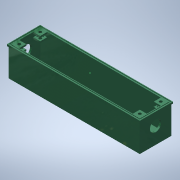
# Autodesk Inventor part: base inferior
Saved by Autodesk Inventor 2021 (Build 250183000, 183)
## iProperties
Created: 2021-03-08
Part Number: base inferior
Material: Steel, Mild, Welded
Document SubType Name: Modeling
Designer: Usuario
Density: 7.85 g/cm^3
Appearance: Smooth - Dark Sea Green
Author: Usuario
Autodesk Inventor part; units mm, degrees
ref_plane "YZ Plane" through (0, 0, 0) normal (1, 0, 0) x (0, 1, 0)
ref_plane "XZ Plane" through (0, 0, 0) normal (0, 1, 0) x (-1, 0, 0)
ref_plane "XY Plane" through (0, 0, 0) normal (0, 0, 1) x (1, 0, 0)
sketch "Sketch1" plane through (0, 0, 0) normal (0, 1, 0) x (-1, 0, 0)
  line L0 (75, -18) -> (-75, -18)
  line L1 (-75, -18) -> (-75, 18)
  line L2 (-75, 18) -> (75, 18)
  line L3 (75, 18) -> (75, -18)
  line L4 (75, -18) -> (-75, 18) construction
  line L5 (-75, -18) -> (75, 18) construction
  point P0 (0, 0)
  dimension "d0" = 150
  dimension "d1" = 36
  constraints: 12 end point, 2 midpoint, 2 parallel, 1 horizontal, 1 perpendicular
  measures "d0" distance of L1.end L2.end
  measures "d1" distance of L0.end L1.end
extrude "Extrusion1" add sketch "Sketch1" along normal blind 2
sketch "Sketch3" plane through (0, 2, 0) normal (0, 1, 0) x (1, 0, 0)
  line L0 (75, 18) -> (-75, 18) projected
  line L1 (-75, 18) -> (-75, -18) projected
  line L2 (73, -16) -> (-73, -16)
  line L3 (-73, -16) -> (-73, 16)
  line L4 (-73, 16) -> (73, 16)
  line L5 (73, 16) -> (73, -16)
  line L6 (-75, -18) -> (75, -18) projected
  line L7 (-75, -18) -> (75, -18)
  line L8 (75, -18) -> (75, 18)
  line L9 (75, 18) -> (-75, 18)
  line L10 (-75, 18) -> (-75, -18)
  point P0 (0, 0)
  constraints: 16 end point, 4 parallel, 2 horizontal, 2 perpendicular
extrude "Extrusion3" add sketch "Sketch3" along normal blind 30
sketch "Sketch4" plane through (-73, 2, 16) normal (1, 0, 0) x (0, 0, -1)
  line L0 (32, 0) -> (0, 0) projected
  line L1 (32, 0) -> (32, 30) projected
  line L2 (0, 30) -> (32, 30) projected
  line L3 (0, 0) -> (0, 30) projected
  line L4 (0, 30) -> (32, 30) projected
  line L5 (32, 0) -> (32, 30) projected
  line L6 (0, 30) -> (32, 30)
  line L7 (32, 30) -> (32, 0)
  line L8 (32, 0) -> (0, 0)
  line L9 (0, 0) -> (0, 30)
  line L10 (32, 0) -> (0, 0) projected
  circle A0 centre (16, 17) radius 6.4
  point P0 (16, -2)
  constraints: 8 end point, 2 parallel, 1 centre point, 1 horizontal, 1 perpendicular
extrude "Extrusion4" cut sketch "Sketch4" against normal blind 30 contours A0
sketch "Sketch5" plane through (73, 2, -16) normal (-1, 0, 0) x (0, 0, 1)
  line L0 (32, 0) -> (0, 0) projected
  line L1 (32, 0) -> (32, 30) projected
  line L2 (0, 30) -> (32, 30) projected
  line L3 (0, 0) -> (0, 30) projected
  line L4 (0, 30) -> (32, 30) projected
  line L5 (0, 30) -> (32, 30)
  line L6 (32, 30) -> (32, 0)
  line L7 (32, 0) -> (0, 0)
  line L8 (0, 0) -> (0, 30)
  line L9 (0, 0) -> (0, 30) projected
  circle A0 centre (16, 17) radius 6.4
  point P0 (16, -2)
  dimension "d23" = 12.8
  constraints: 8 end point, 2 parallel, 1 centre point, 1 horizontal, 1 perpendicular
  measures "d23" diameter of A0
extrude "Extrusion5" cut sketch "Sketch5" against normal blind 30 contours A0
sketch "Sketch6" plane through (0, 32, 0) normal (0, 1, 0) x (1, 0, 0)
  line L0 (75, 18) -> (-75, 18) projected
  line L1 (-75, 18) -> (-75, -18) projected
  line L2 (-75, -18) -> (75, -18) projected
  line L3 (75, -18) -> (75, 18) projected
  line L4 (73, -16) -> (-73, -16) projected
  line L5 (-73, -16) -> (-73, 16) projected
  line L6 (-73, 16) -> (73, 16) projected
  line L7 (73, 16) -> (73, -16) projected
  line L8 (-76, -18) -> (-76, -19)
  line L9 (75, -18) -> (75, 18) projected
  line L10 (75, 19) -> (76, 19)
  line L11 (76, 19) -> (-76, 19)
  line L12 (-76, 19) -> (-76, -19)
  line L13 (-76, -19) -> (76, -19)
  line L14 (76, -19) -> (76, 19)
  line L15 (-73, -16) -> (-73, 16) projected
  line L16 (73, 16) -> (-73, 16) projected
  line L17 (-73, -16) -> (73, -16)
  line L18 (73, -16) -> (73, 16)
  line L19 (73, 16) -> (-73, 16)
  line L20 (-73, 16) -> (-73, -16)
  point P0 (0, 0)
  dimension "d26" = 1
  dimension "d27" = 1
  dimension "d28" = 1
  dimension "d29" = 1
  constraints: 20 end point, 4 parallel, 2 horizontal, 2 perpendicular
  measures "d26" distance of L1.end L8.start
  measures "d27" distance of L8.start L8.end
  measures "d28" distance of L0.start L10.start
  measures "d29" distance of L10.start L10.end
extrude "Extrusion6" add sketch "Sketch6" along normal blind 2 contours L3 L2 L1 L0 | L12 L11 L10 L14 L13 L8
sketch "Sketch7" plane through (0, 34, 0) normal (0, 1, 0) x (1, 0, 0)
  line L0 (76, 19) -> (-76, 19) projected
  line L1 (-76, 19) -> (-76, -19) projected
  line L2 (-76, -19) -> (76, -19) projected
  line L3 (76, -19) -> (76, 19) projected
  line L4 (73, 16) -> (73, -16) projected
  line L5 (73, -16) -> (-73, -16) projected
  line L6 (-73, -16) -> (-73, 16) projected
  line L7 (-73, 16) -> (73, 16) projected
  line L8 (73, -16) -> (-73, -16) projected
  line L9 (-73.85, -16) -> (-73.85, -16.85)
  line L10 (-76, 19) -> (-76, -19) projected
  line L11 (-76, -19) -> (-76, -18.15)
  line L12 (76, 19) -> (-76, 19) projected
  line L13 (76, 19) -> (75.15, 19)
  line L14 (-73, 16) -> (73, 16) projected
  line L15 (73, 16.85) -> (73.85, 16.85)
  line L16 (73.85, 16.85) -> (-73.85, 16.85)
  line L17 (-73.85, 16.85) -> (-73.85, -16.85)
  line L18 (-73.85, -16.85) -> (73.85, -16.85)
  line L19 (73.85, -16.85) -> (73.85, 16.85)
  line L20 (-75.15, -18.15) -> (75.15, -18.15)
  line L21 (75.15, -18.15) -> (75.15, 18.15)
  line L22 (75.15, 18.15) -> (-75.15, 18.15)
  line L23 (-75.15, 18.15) -> (-75.15, -18.15)
  point P0 (0, 0)
  dimension "d34" = 0.85
  constraints: 24 end point, 4 parallel, 2 horizontal, 2 perpendicular, 2 point on line
  measures "d34" distance of L1.end L11.end
extrude "Extrusion7" cut sketch "Sketch7" against normal blind 0.75 contours L23 L22 L21 L20
sketch "Sketch8" plane through (0, 34, 0) normal (0, 1, 0) x (1, 0, 0)
  point P0 (0, 0)
sketch "Sketch9" plane through (-73, 2, 16) normal (1, 0, 0) x (0, 0, -1)
  point P0 (16, -2)
sketch "Sketch29" plane through (0, 34, 0) normal (0, 1, 0) x (1, 0, 0)
  line L0 (-73.85, -16.85) -> (73.85, -16.85) projected
  line L1 (73.85, -16.85) -> (73.85, 16.85) projected
  line L2 (73.85, 16.85) -> (-73.85, 16.85) projected
  line L3 (-73.85, 16.85) -> (-73.85, -16.85) projected
  line L4 (73, 16) -> (73, -16) projected
  line L5 (73, -16) -> (-73, -16) projected
  line L6 (-73, -16) -> (-73, 16) projected
  line L7 (-73, 16) -> (73, 16) projected
  line L8 (75.15, 18.15) -> (75.15, -18.15) projected
  line L9 (-75.15, 18.15) -> (75.15, 18.15) projected
  line L10 (-75.15, -18.15) -> (-75.15, 18.15) projected
  line L11 (75.15, -18.15) -> (-75.15, -18.15) projected
  line L12 (73.85, -16.85) -> (73.85, 16.85) projected
  line L13 (-73.85, -16.85) -> (73.85, -16.85) projected
  line L14 (-73.85, 16.85) -> (-73.85, -16.85) projected
  line L15 (73.85, 16.85) -> (-73.85, 16.85) projected
  line L16 (-76, 19) -> (-76, -19) projected
  line L17 (76, 19) -> (-76, 19) projected
  line L18 (-76, 19) -> (-76, -19) projected
  line L19 (-76, -19) -> (76, -19) projected
  line L20 (76, -19) -> (76, 19) projected
  line L21 (-75.15, 18.15) -> (75.15, 18.15) projected
  line L22 (75.15, 18.15) -> (75.15, -18.15) projected
  line L23 (75.15, -18.15) -> (-75.15, -18.15) projected
  line L24 (-75.15, -18.15) -> (-75.15, 18.15) projected
  line L25 (-73, -16) -> (73, -16) projected
  line L26 (-73, -16) -> (-73, 16) projected
  line L27 (-73, -16) -> (-65.5, -16) construction
  line L28 (-73, -16) -> (-65, -16)
  line L29 (-65, -16) -> (-65, -8)
  line L30 (-65, -8) -> (-73, -8)
  line L31 (-73, -8) -> (-73, -16)
  line L32 (-73, 16) -> (-65, 16)
  line L33 (-65, 16) -> (-65, 8)
  line L34 (-65, 8) -> (-73, 8)
  line L35 (-73, 8) -> (-73, 16)
  line L36 (73, 16) -> (-73, 16) projected
  line L37 (73, 16) -> (65, 16)
  line L38 (65, 16) -> (65, 8)
  line L39 (65, 8) -> (73, 8)
  line L40 (73, 8) -> (73, 16)
  line L41 (73, -16) -> (65, -16)
  line L42 (65, -16) -> (65, -8)
  line L43 (65, -8) -> (73, -8)
  line L44 (73, -8) -> (73, -16)
  point P0 (0, 0)
  dimension "d120" = 8
  dimension "d121" = 8
  dimension "d122" = 8
  dimension "d123" = 8
  dimension "d124" = 8
  dimension "d125" = 8
  dimension "d126" = 8
  dimension "d127" = 8
  constraints: 34 end point, 8 parallel, 5 horizontal, 4 perpendicular
  measures "d120" distance of L30.end L29.end
  measures "d121" distance of L29.end L28.end
  measures "d122" distance of L33.end L34.end
  measures "d123" distance of L32.end L33.end
  measures "d124" distance of L39.end L38.end
  measures "d125" distance of L38.end L37.end
  measures "d126" distance of L42.end L43.end
  measures "d127" distance of L41.end L42.end
extrude "Extrusion22" add sketch "Sketch29" against normal blind 7 contours L4 L39 L38 L7 | L4 L5 L42 L43 | L33 L34 L6 L7 | L5 L6 L30 L29
sketch "Sketch30" plane through (-65, 34, -8) normal (1, 0, 0) x (0, 0, -1)
  line L0 (0, 0) -> (8, 0) projected
  line L1 (0, 0) -> (0, -7) projected
  line L2 (8, -7) -> (0, -7) projected
  line L3 (8, 0) -> (8, -7) projected
  line L4 (-24, 0) -> (-16, 0) projected
  line L5 (-24, -7) -> (-24, 0) projected
  line L6 (-16, -7) -> (-24, -7) projected
  line L7 (-16, 0) -> (-16, -7) projected
  line L8 (0, 0) -> (0, -7) projected
  line L9 (8, 0) -> (0, 0)
  line L10 (0, 0) -> (0, -1.8)
  line L11 (0, -1.8) -> (8, -1.8)
  line L12 (8, -1.8) -> (8, 0)
  line L13 (8, 0) -> (8, -7) projected
  line L14 (8, -7) -> (0, -7)
  line L15 (0, -7) -> (0, -5.2)
  line L16 (0, -5.2) -> (8, -5.2)
  line L17 (8, -5.2) -> (8, -7)
  line L18 (0, -1.8) -> (8, -1.8)
  line L19 (8, -1.8) -> (8, -5.2)
  line L20 (8, -5.2) -> (0, -5.2)
  line L21 (0, -5.2) -> (0, -1.8)
  line L22 (-24, 0) -> (-16, 0) projected
  line L23 (-16, 0) -> (-24, 0)
  line L24 (-24, 0) -> (-24, -1.8)
  line L25 (-24, -1.8) -> (-16, -1.8)
  line L26 (-16, -1.8) -> (-16, 0)
  line L27 (-16, -7) -> (-24, -7)
  line L28 (-24, -7) -> (-24, -5.2)
  line L29 (-24, -5.2) -> (-16, -5.2)
  line L30 (-16, -5.2) -> (-16, -7)
  line L31 (-16, -1.8) -> (-24, -1.8)
  line L32 (-24, -1.8) -> (-24, -5.2)
  line L33 (-24, -5.2) -> (-16, -5.2)
  line L34 (-16, -5.2) -> (-16, -1.8)
  point P0 (-8, -34)
  point P1 (-24, -5.2)
  point P2 (-16, -5.2)
  point P3 (-16, -1.8)
  point P4 (-24, -1.8)
  point P5 (0, -5.2)
  point P6 (8, -5.2)
  point P7 (8, -1.8)
  point P8 (0, -1.8)
  dimension "d130" = 1.8
  dimension "d131" = 1.8
  dimension "d132" = 8
  dimension "d133" = 1.8
  dimension "d134" = 8
  dimension "d135" = 1.8
  constraints: 48 end point, 12 parallel, 6 horizontal, 6 perpendicular, 2 point on line
  measures "d130" distance of L10.end L9.end
  measures "d131" distance of L14.end L15.end
  measures "d132" distance of L25.end L24.end
  measures "d133" distance of L24.end L23.end
  measures "d134" distance of L28.end L29.end
  measures "d135" distance of L27.end L28.end
extrude "Extrusion23" cut sketch "Sketch30" against normal blind 8 contours L11 L3 L16 L1 | L25 L7 L29 L5
sketch "Sketch31" plane through (65, 34, -16) normal (-1, 0, 0) x (0, 0, 1)
  point P0 (16, -34)
sketch "Sketch32" plane through (65, 34, -16) normal (-1, 0, 0) x (0, 0, 1)
  line L0 (0, 0) -> (8, 0) projected
  line L1 (0, -7) -> (0, 0) projected
  line L2 (8, -7) -> (0, -7) projected
  line L3 (8, 0) -> (8, -7) projected
  line L4 (32, -7) -> (24, -7) projected
  line L5 (24, 0) -> (32, 0) projected
  line L6 (24, 0) -> (24, -7) projected
  line L7 (32, -7) -> (24, -7) projected
  line L8 (32, 0) -> (32, -7) projected
  line L9 (0, 0) -> (8, 0)
  line L10 (8, 0) -> (8, -1.8)
  line L11 (8, -1.8) -> (0, -1.8)
  line L12 (0, -1.8) -> (0, 0)
  line L13 (8, -7) -> (0, -7)
  line L14 (0, -7) -> (0, -5.2)
  line L15 (0, -5.2) -> (8, -5.2)
  line L16 (8, -5.2) -> (8, -7)
  line L17 (0, -1.8) -> (8, -1.8)
  line L18 (8, -1.8) -> (8, -5.2)
  line L19 (8, -5.2) -> (0, -5.2)
  line L20 (0, -5.2) -> (0, -1.8)
  line L21 (24, 0) -> (32, 0) projected
  line L22 (24, 0) -> (32, 0)
  line L23 (32, 0) -> (32, -1.8)
  line L24 (32, -1.8) -> (24, -1.8)
  line L25 (24, -1.8) -> (24, 0)
  line L26 (24, -7) -> (32, -7)
  line L27 (32, -7) -> (32, -5.2)
  line L28 (32, -5.2) -> (24, -5.2)
  line L29 (24, -5.2) -> (24, -7)
  line L30 (24, -1.8) -> (32, -1.8)
  line L31 (32, -1.8) -> (32, -5.2)
  line L32 (32, -5.2) -> (24, -5.2)
  line L33 (24, -5.2) -> (24, -1.8)
  point P0 (16, -34)
  point P1 (24, -5.2)
  point P2 (32, -5.2)
  point P3 (32, -1.8)
  point P4 (24, -1.8)
  point P5 (0, -5.2)
  point P6 (8, -5.2)
  point P7 (8, -1.8)
  point P8 (0, -1.8)
  dimension "d138" = 8
  dimension "d139" = 1.8
  dimension "d140" = 8
  dimension "d141" = 1.8
  dimension "d142" = 8
  dimension "d143" = 1.8
  dimension "d144" = 8
  dimension "d145" = 1.8
  constraints: 48 end point, 12 parallel, 6 horizontal, 6 perpendicular
  measures "d138" distance of L10.end L11.end
  measures "d139" distance of L9.end L10.end
  measures "d140" distance of L14.end L15.end
  measures "d141" distance of L13.end L14.end
  measures "d142" distance of L23.end L24.end
  measures "d143" distance of L22.end L23.end
  measures "d144" distance of L28.end L27.end
  measures "d145" distance of L27.end L26.end
extrude "Extrusion24" cut sketch "Sketch32" against normal blind 8 contours L11 L3 L15 L1 | L28 L6 L24 L8
sketch "Sketch34" plane through (65, 28.8, -8) normal (0, 1, 0) x (1, 0, 0)
  line L0 (8, 8) -> (0, 8)
  line L1 (0, 8) -> (0, 0)
  line L2 (0, 0) -> (8, 0)
  line L3 (8, 0) -> (8, 8)
  line L4 (0, 0) -> (0, 8)
  line L5 (8, 0) -> (0, 0) projected
  circle A0 centre (4, 4) radius 3.35
  line L6 (1.6312, 1.6312) -> (0.7641, 4.867)
  line L7 (0.7641, 4.867) -> (3.133, 7.2359)
  line L8 (3.133, 7.2359) -> (6.3688, 6.3688)
  line L9 (6.3688, 6.3688) -> (7.2359, 3.133)
  line L10 (7.2359, 3.133) -> (4.867, 0.7641)
  line L11 (4.867, 0.7641) -> (1.6312, 1.6312)
  point P0 (-65, -8)
  constraints: 22 end point, 2 parallel, 1 coincident, 1 horizontal, 1 perpendicular, 16 other
sketch "Sketch35" plane through (65, 28.8, 16) normal (0, 1, 0) x (1, 0, 0)
  line L0 (8, 8) -> (0, 8)
  line L1 (0, 8) -> (0, 0)
  line L2 (0, 0) -> (8, 0)
  line L3 (8, 0) -> (8, 8)
  line L4 (0, 0) -> (0, 8)
  line L5 (8, 0) -> (8, 8) projected
  line L6 (0, 0) -> (0, 8) projected
  circle A0 centre (4, 4) radius 3.35
  line L7 (1.6312, 1.6312) -> (0.7641, 4.867)
  line L8 (0.7641, 4.867) -> (3.133, 7.2359)
  line L9 (3.133, 7.2359) -> (6.3688, 6.3688)
  line L10 (6.3688, 6.3688) -> (7.2359, 3.133)
  line L11 (7.2359, 3.133) -> (4.867, 0.7641)
  line L12 (4.867, 0.7641) -> (1.6312, 1.6312)
  point P0 (-65, 16)
  constraints: 22 end point, 2 parallel, 1 coincident, 1 horizontal, 1 perpendicular, 1 point on line, 16 other
extrude "Extrusion26" cut sketch "Sketch35" against normal blind 1 contours L10 L11 L12 L7 L8 L9
extrude "Extrusion27" cut sketch "Sketch34" against normal blind 1 contours L9 L10 L11 L6 L7 L8
sketch "Sketch36" plane through (-65, 28.8, -8) normal (0, 1, 0) x (1, 0, 0)
  line L0 (-8, 8) -> (0, 8)
  line L1 (0, 8) -> (0, 0)
  line L2 (0, 0) -> (-8, 0)
  line L3 (-8, 0) -> (-8, 8)
  line L4 (0, 0) -> (-8, 0)
  circle A0 centre (-4, 4) radius 3.35
  line L5 (-1.6312, 1.6312) -> (-4.867, 0.7641)
  line L6 (-4.867, 0.7641) -> (-7.2359, 3.133)
  line L7 (-7.2359, 3.133) -> (-6.3688, 6.3688)
  line L8 (-6.3688, 6.3688) -> (-3.133, 7.2359)
  line L9 (-3.133, 7.2359) -> (-0.7641, 4.867)
  line L10 (-0.7641, 4.867) -> (-1.6312, 1.6312)
  point P0 (65, -8)
  dimension "d163" = 6.7
  constraints: 22 end point, 2 parallel, 1 coincident, 1 horizontal, 1 perpendicular, 1 point on line, 16 other
extrude "Extrusion28" cut sketch "Sketch36" against normal blind 1 contours L10 L5 L6 L7 L8 L9
sketch "Sketch37" plane through (-73, 28.8, 8) normal (0, 1, 0) x (1, 0, 0)
  line L0 (0, 0) -> (8, 0) projected
  line L1 (8, 0) -> (8, -8) projected
  line L2 (0, 0) -> (8, 0)
  line L3 (8, 0) -> (8, -8)
  line L4 (8, -8) -> (0, -8)
  line L5 (0, -8) -> (0, 0)
  circle A0 centre (4, -4) radius 3.35
  line L6 (6.3688, -6.3688) -> (3.133, -7.2359)
  line L7 (3.133, -7.2359) -> (0.7641, -4.867)
  line L8 (0.7641, -4.867) -> (1.6312, -1.6312)
  line L9 (1.6312, -1.6312) -> (4.867, -0.7641)
  line L10 (4.867, -0.7641) -> (7.2359, -3.133)
  line L11 (7.2359, -3.133) -> (6.3688, -6.3688)
  point P0 (73, 8)
  dimension "d166" = 6.7
  constraints: 20 end point, 2 parallel, 1 coincident, 1 horizontal, 1 perpendicular, 16 other
extrude "Extrusion29" cut sketch "Sketch37" against normal blind 1 contours L11 L6 L7 L8 L9 L10
sketch "Sketch38" plane through (0, 34, 0) normal (0, 1, 0) x (1, 0, 0)
  line L0 (-73.85, -16.85) -> (73.85, -16.85) projected
  line L1 (73.85, -16.85) -> (73.85, 16.85) projected
  line L2 (73.85, 16.85) -> (-73.85, 16.85) projected
  line L3 (-73.85, 16.85) -> (-73.85, -16.85) projected
  line L4 (73, 8) -> (73, -8) projected
  line L5 (73, -8) -> (65, -8) projected
  line L6 (65, -8) -> (65, -16) projected
  line L7 (65, -16) -> (-65, -16) projected
  line L8 (-65, -16) -> (-65, -8) projected
  line L9 (-65, -8) -> (-73, -8) projected
  line L10 (-73, -8) -> (-73, 8) projected
  line L11 (-73, 8) -> (-65, 8) projected
  line L12 (-65, 8) -> (-65, 16) projected
  line L13 (-65, 16) -> (65, 16) projected
  line L14 (65, 16) -> (65, 8) projected
  line L15 (65, 8) -> (73, 8) projected
  line L16 (-65, 8) -> (-73, 8) projected
  line L17 (-65, 8) -> (-73, 8)
  line L18 (-73, 8) -> (-73, 16)
  line L19 (-73, 16) -> (-65, 16)
  line L20 (-65, 16) -> (-65, 8)
  circle A0 centre (-69, 12) radius 1.65
  line L21 (-73, -8) -> (-65, -8) projected
  line L22 (-65, -8) -> (-73, -8)
  line L23 (-73, -8) -> (-73, -16)
  line L24 (-73, -16) -> (-65, -16)
  line L25 (-65, -16) -> (-65, -8)
  circle A1 centre (-69, -12) radius 1.65
  line L26 (73, 8) -> (65, 8) projected
  line L27 (65, 8) -> (73, 8)
  line L28 (73, 8) -> (73, 16)
  line L29 (73, 16) -> (65, 16)
  line L30 (65, 16) -> (65, 8)
  line L31 (65, -8) -> (65, -16) projected
  line L32 (65, -8) -> (73, -8)
  line L33 (73, -8) -> (73, -16)
  line L34 (73, -16) -> (65, -16)
  line L35 (65, -16) -> (65, -8)
  circle A2 centre (69, 12) radius 1.65
  circle A3 centre (69, -12) radius 1.65
  point P0 (0, 0)
  dimension "d169" = 8
  dimension "d170" = 8
  dimension "d171" = 3.3
  dimension "d172" = 8
  dimension "d173" = 8
  dimension "d174" = 3.3
  dimension "d175" = 8
  dimension "d176" = 8
  dimension "d177" = 8
  dimension "d178" = 8
  dimension "d179" = 3.3
  dimension "d180" = 3.3
  constraints: 32 end point, 8 parallel, 4 centre point, 4 horizontal, 4 perpendicular
  measures "d169" distance of L18.end L19.end
  measures "d170" distance of L17.end L18.end
  measures "d171" diameter of A0
  measures "d172" distance of L24.end L23.end
  measures "d173" distance of L23.end L22.end
  measures "d174" diameter of A1
  measures "d175" distance of L29.end L28.end
  measures "d176" distance of L28.end L27.end
  measures "d177" distance of L33.end L34.end
  measures "d178" distance of L32.end L33.end
  measures "d179" diameter of A2
  measures "d180" diameter of A3
extrude "Extrusion30" cut sketch "Sketch38" against normal blind 8 contours A0 | A1 | A2 | A3
body "Solid1"
